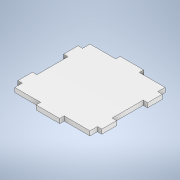
# Autodesk Inventor part: Inferior
Saved by Autodesk Inventor 2020.2 (Build 242310000, 310)
## iProperties
Created: 2020-03-18
Part Number: Inferior
Material: LCP Plastic
Document SubType Name: Modeling
Designer: ARQ SEVILLA R
Density: 1.626 g/cm^3
Appearance: Smooth - White
Author: ARQ SEVILLA R
Autodesk Inventor part; units mm, degrees
ref_plane "YZ Plane" through (0, 0, 0) normal (1, 0, 0) x (0, 1, 0)
ref_plane "XZ Plane" through (0, 0, 0) normal (0, 1, 0) x (-1, 0, 0)
ref_plane "XY Plane" through (0, 0, 0) normal (0, 0, 1) x (1, 0, 0)
sketch "Sketch1" plane through (0, 0, 0) normal (0, 1, 0) x (-1, 0, 0)
  line L0 (-28.5, -57) -> (-28.5, -28.5) construction
  line L1 (-28.5, -28.5) -> (-57, -28.5) construction
  line L2 (0, -49) -> (-3, -49)
  line L3 (-3, -49) -> (-3, -57)
  line L4 (0, -49) -> (0, -39)
  line L5 (0, -39) -> (-3, -39)
  line L6 (-3, -39) -> (-3, -28.5)
  line L7 (0, -8) -> (-3, -8)
  line L8 (-3, -8) -> (-3, 0)
  line L9 (0, -18) -> (-3, -18)
  line L10 (-3, -18) -> (-3, -28.5)
  line L11 (0, -8) -> (0, -18)
  line L12 (0, -39) -> (0, -49)
  line L13 (0, -49) -> (0, -39)
  line L14 (0, -18) -> (0, -8)
  line L15 (-57, -49) -> (-54, -49)
  line L16 (-54, -49) -> (-54, -57)
  line L17 (-57, -49) -> (-57, -39)
  line L18 (-57, -39) -> (-54, -39)
  line L19 (-54, -39) -> (-54, -28.5)
  line L20 (-57, -8) -> (-54, -8)
  line L21 (-54, -8) -> (-54, 0)
  line L22 (-57, -18) -> (-54, -18)
  line L23 (-54, -18) -> (-54, -28.5)
  line L24 (-57, -8) -> (-57, -18)
  line L25 (-57, -39) -> (-57, -49)
  line L26 (-57, -49) -> (-57, -39)
  line L27 (-57, -18) -> (-57, -8)
  line L28 (-57, -49) -> (-57, -39)
  line L29 (-57, -18) -> (-57, -8)
  line L30 (-28.5, -54) -> (-36.5, -54)
  line L31 (-36.5, -54) -> (-36.5, -57)
  line L32 (-28.5, -54) -> (-20.5, -54)
  line L33 (-20.5, -54) -> (-20.5, -57)
  line L34 (-3, -57) -> (-20.5, -57)
  line L35 (-36.5, -57) -> (-54, -57)
  line L36 (-28.5, -3) -> (-36.5, -3)
  line L37 (-36.5, -3) -> (-36.5, 0)
  line L38 (-20.5, -3) -> (-20.5, 0)
  line L39 (-28.5, -3) -> (-20.5, -3)
  line L40 (-54, 0) -> (-36.5, 0)
  line L41 (-20.5, 0) -> (-3, 0)
  point P0 (0, 0)
  point P1 (0, -57)
  dimension "d3" = 3
  dimension "d4" = 10
  dimension "d5" = 3
  dimension "d6" = 3
  dimension "d7" = 8
  constraints: 84 end point, 24 symmetric about line, 14 perpendicular, 3 vertical, 2 horizontal, 1 point on line
  measures "d3" distance of L2.start L2.end
  measures "d4" distance of L2.start L4.end
  measures "d5" distance of L4.end L5.end
  measures "d6" distance of L0.start L30.start
  measures "d7" distance of L30.start L30.end
extrude "Extrusion1" add sketch "Sketch1" along normal blind 3
sketch "Sketch2" plane through (0, 3, 0) normal (0, 1, 0) x (1, 0, 0)
  line L0 (36.5, 0) -> (54, 0) projected
  line L1 (36.5, 3) -> (36.5, 0) projected
  line L2 (36.5, 0) -> (36.5, 3)
  line L3 (36.5, 3) -> (54, 3)
  line L4 (54, 0) -> (54, 8) projected
  line L5 (20.5, 0) -> (20.5, 3) projected
  line L6 (20.5, 0) -> (20.5, 3)
  line L7 (20.5, 3) -> (36.5, 3) projected
  line L8 (20.5, 3) -> (36.5, 3)
  line L9 (36.5, 3) -> (36.5, 0)
  line L10 (3, 0) -> (20.5, 0) projected
  line L11 (20.5, 0) -> (20.5, 3)
  line L12 (3, 0) -> (3, 3)
  line L13 (3, 8) -> (3, 0) projected
  line L14 (20.5, 3) -> (3, 3)
  point P0 (0, 0)
  constraints: 16 end point, 4 collinear, 3 perpendicular, 2 point on line
extrude "Extrusion2" cut sketch "Sketch2" against normal up to surface (3 mm away)
sketch "Sketch3" plane through (0, 3, 0) normal (0, 1, 0) x (1, 0, 0)
  line L0 (3, 3) -> (20.5, 3)
  line L1 (3, 3) -> (54, 3) projected
  line L2 (20.5, 3) -> (20.5, 0)
  line L3 (36.5, 54) -> (20.5, 54) projected
  line L4 (28.5, 54) -> (28.5, 14.4088) construction
  line L5 (54, 3) -> (36.5, 3)
  line L6 (36.5, 3) -> (36.5, 0)
  line L7 (20.5, 0) -> (36.5, 0)
  point P0 (0, 0)
  dimension "d12" = 17.5
  constraints: 12 end point, 2 symmetric about line, 1 horizontal, 1 midpoint, 1 perpendicular, 1 point on line, 1 vertical
  measures "d12" distance of L0.start L0.end
extrude "Extrusion3" add sketch "Sketch3" against normal up to surface (3 mm away)
sketch "Sketch4" plane through (0, 3, 0) normal (0, 1, 0) x (1, 0, 0)
  line L0 (36.5, 54) -> (20.5, 54) projected
  line L1 (20.5, 54) -> (3, 54)
  line L2 (3, 57) -> (3, 49) projected
  line L3 (36.5, 57) -> (36.5, 54) projected
  line L4 (36.5, 54) -> (54, 54)
  line L5 (54, 49) -> (54, 57) projected
  line L6 (20.5, 57) -> (3, 57) projected
  line L7 (3, 54) -> (3, 57)
  line L8 (3, 57) -> (20.5, 57)
  line L9 (20.5, 57) -> (20.5, 54)
  line L10 (36.5, 57) -> (36.5, 54)
  line L11 (54, 57) -> (36.5, 57) projected
  line L12 (36.5, 57) -> (54, 57)
  line L13 (54, 57) -> (54, 54)
  point P0 (0, 0)
  constraints: 16 end point, 3 perpendicular, 3 point on line, 2 equal length, 1 horizontal, 1 vertical
extrude "Extrusion4" cut sketch "Sketch4" against normal up to surface (3 mm away)
sketch "Sketch5" plane through (0, 3, 0) normal (0, 1, 0) x (1, 0, 0)
  line L0 (54, 18) -> (54, 39) projected
  line L1 (54, 28.5) -> (3, 28.5) construction
  line L2 (3, 39) -> (3, 18) projected
  line L3 (3, 3) -> (20.5, 3) projected
  line L4 (3, 3) -> (20.5, 3)
  line L5 (20.5, 3) -> (20.5, 0)
  line L6 (20.5, 0) -> (36.5, 0) projected
  line L7 (20.5, 0) -> (36.5, 0)
  line L8 (36.5, 0) -> (36.5, 3)
  line L9 (36.5, 3) -> (54, 3) projected
  line L10 (36.5, 3) -> (54, 3)
  line L11 (3, 54) -> (20.5, 54)
  line L12 (20.5, 54) -> (20.5, 57)
  line L13 (20.5, 57) -> (36.5, 57)
  line L14 (36.5, 57) -> (36.5, 54)
  line L15 (36.5, 54) -> (54, 54)
  line L16 (20.5, 54) -> (36.5, 54)
  line L17 (54, 54) -> (3, 54) projected
  point P0 (0, 0)
  constraints: 24 end point, 6 symmetric about line, 3 collinear, 2 midpoint, 2 perpendicular, 1 horizontal, 1 point on line
extrude "Extrusion5" add sketch "Sketch5" against normal up to surface (3 mm away)
body "Solid1"
